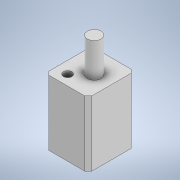
# Autodesk Inventor part: pneumaticActuator
Saved by Autodesk Inventor 2021 (Build 250183000, 183)
## iProperties
Created: 2021-01-06
Part Number: pneumaticActuator
Material: Generic
Document SubType Name: Modeling
Designer: awitc
Density: 1 g/cm^3
Appearance: Default
Author: awitc
Autodesk Inventor part; units mm, degrees
ref_plane "YZ Plane" through (0, 0, 0) normal (1, 0, 0) x (0, 1, 0)
ref_plane "XZ Plane" through (0, 0, 0) normal (0, 1, 0) x (-1, 0, 0)
ref_plane "XY Plane" through (0, 0, 0) normal (0, 0, 1) x (1, 0, 0)
sketch "Sketch4" plane through (0, 0, 0) normal (0, 1, 0) x (-1, 0, 0)
  line L0 (0, 0) -> (25, 0)
  line L1 (25, 0) -> (25, -27)
  line L2 (25, -27) -> (0, -27)
  line L3 (0, -27) -> (0, 0)
  line L4 (25, 0) -> (18, 0)
  circle A0 centre (18, -6) radius 2.5
  circle A1 centre (18, -21) radius 2.5
  dimension "d35" = 25
  dimension "d36" = 27
  dimension "d39" = 5
  dimension "d41" = 5
  constraints: 10 end point, 2 centre point, 2 parallel, 1 horizontal, 1 perpendicular, 1 point on line
  measures "d35" distance of L1.end L2.end
  measures "d36" distance of L0.end L1.end
  measures "d39" diameter of A0
  measures "d41" diameter of A1
extrude "Extrusion4" add sketch "Sketch4" along normal blind 38
sketch "Sketch5" plane through (0, 38, 0) normal (0, 1, 0) x (1, 0, 0)
  line L0 (0, 0) -> (0, 27) projected
  line L1 (0, 0) -> (0, 27)
  line L2 (0, 27) -> (0, 13.5)
  line L3 (0, 13.5) -> (-10, 13.5)
  circle A0 centre (-10, 13.5) radius 4
  dimension "d44" = 10
  dimension "d51" = 8
  constraints: 6 end point, 1 centre point, 1 collinear, 1 midpoint, 1 perpendicular
  measures "d44" distance of L2.end L3.end
  measures "d51" diameter of A0
extrude "Extrusion5" add sketch "Sketch5" along normal blind 20
chamfer "Chamfer2" distance 2 angle 45 4 edges at (-25, 19, 0) (-25, 19, -27) (0, 19, -27) (0, 19, 0)
body "Solid2"
